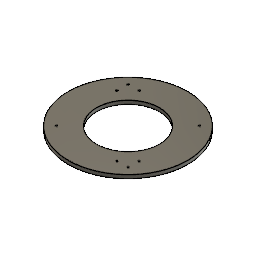
bot_joint_print v4 (Autodesk Fusion 360 design; units mm, degrees)
Autodesk Fusion 360 part; units mm, degrees
sketch "Sketch1" plane through (0, 0, 0) normal (0, 1, 0) x (1, 0, 0)
  circle A0 centre (0, 0) radius 17.095
  circle A1 centre (0, 0) radius 32.5
  line L0 (-21.05, 0) -> (0, 0)
  line L1 (0, 0) -> (-19.4454, 19.4454)
  circle A2 centre (-19.4454, 19.4454) radius 0.5
  circle A3 centre (-19.4454, -19.4454) radius 0.5
  circle A4 centre (19.4454, -19.4454) radius 0.5
  circle A5 centre (19.4454, 19.4454) radius 0.5
  line L2 (17.3241, -8.1317) -> (8.1317, -17.3241)
  line L3 (0, 0) -> (12.7279, -12.7279)
  line L4 (10.253, -19.4454) -> (8.1317, -17.3241)
  line L5 (8.1317, -17.3241) -> (11.3137, -14.1421)
  line L6 (11.3137, -14.1421) -> (13.435, -16.2635)
  line L7 (13.435, -16.2635) -> (10.253, -19.4454)
  line L8 (19.4454, -10.253) -> (17.3241, -8.1317)
  line L9 (17.3241, -8.1317) -> (14.1421, -11.3137)
  line L10 (14.1421, -11.3137) -> (16.2635, -13.435)
  line L11 (16.2635, -13.435) -> (19.4454, -10.253)
  line L12 (11.844, -17.8544) -> (13.6118, -19.6222)
  circle A6 centre (13.6118, -19.6222) radius 0.5
  line L13 (17.8544, -11.844) -> (19.6222, -13.6118)
  circle A7 centre (19.6222, -13.6118) radius 0.5
  circle A8 centre (-13.6118, 19.6222) radius 0.5
  circle A9 centre (-19.6222, 13.6118) radius 0.5
  dimension "d1" = 34.19
  dimension "d4" = 21.05
  dimension "d7" = 27.5
  dimension "d8" = 1
  dimension "d9" = 45
  dimension "d13" = 13
  dimension "d14" = 18
  dimension "d15" = 3
  dimension "d16" = 4.5
  dimension "d18" = 4.5
  dimension "d19" = 2.5
  dimension "d20" = 1
  dimension "d21" = 2.5
  dimension "d22" = 1
  dimension "d24" = 360
  dimension "d27" = 65
  measures "d1" diameter of A0
  measures "d4" distance of L0.start A0.centre
  measures "d7" distance of A0.centre L1.end
  measures "d8" diameter of A2
  measures "d9" angle of L0 L1
  measures "d13" distance of L2.start L2.end
  measures "d14" distance of A0.centre L3.end
  measures "d15" distance of L2.end L4.start
  measures "d16" distance of L4.start L6.end
  measures "d18" distance of L8.start L10.end
  measures "d19" distance of L12.start L12.end
  measures "d20" diameter of A6
  measures "d21" distance of L13.start L13.end
  measures "d22" diameter of A7
  measures "d27" diameter of A1
extrude "Extrude1" add sketch "Sketch1" along normal blind 2 contours A1 | L2 L8 L9 L10 L11 | L2 L4 L5 L6 L7
